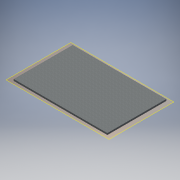
# Autodesk Inventor part: Zwischendecke
Saved by Autodesk Inventor 2017 (Build 210142000, 142)
## iProperties
Created: 2017-06-01
Part Number: Zwischendecke
Material: Beton
Document SubType Name: Modeling
Designer: Fake
Density: 2.40731 g/cm^3
Appearance: Waschbeton - warm-grau
Author: Fake
Autodesk Inventor part; units mm, degrees
ref_plane "YZ Plane" through (0, 0, 0) normal (1, 0, 0) x (0, 1, 0)
ref_plane "XZ Plane" through (0, 0, 0) normal (0, 1, 0) x (-1, 0, 0)
ref_plane "XY Plane" through (0, 0, 0) normal (0, 0, 1) x (1, 0, 0)
ref_plane "Arbeitsebene1" through (-317.6174, -149.9495, 3700) normal (0, 0, 1) x (1, 0, 0)
sketch "Skizze1" plane through (-317.6174, -149.9495, 3700) normal (0, 0, 1) x (1, 0, 0)
  line L0 (5797.6174, 3524.9495) -> (5797.6174, -3225.0505) projected
  line L1 (5797.6174, -3225.0505) -> (-3682.3826, -3225.0505) projected
  line L2 (-3682.3826, -3225.0505) -> (-3682.3826, -1925.0505) projected
  line L3 (-3682.3826, -1925.0505) -> (-5162.3826, -1925.0505) projected
  line L4 (-5162.3826, -1925.0505) -> (-5162.3826, 3524.9495) projected
  line L5 (-5162.3826, 3524.9495) -> (5797.6174, 3524.9495) projected
  line L6 (-5162.3826, -3425.0505) -> (-5162.3826, -2125.0505) projected
  line L7 (-5162.3826, -2125.0505) -> (-3882.3826, -2125.0505) projected
  line L8 (-3882.3826, -2125.0505) -> (-3882.3826, -3425.0505) projected
  line L9 (-3882.3826, -3425.0505) -> (5997.6174, -3425.0505) projected
  line L10 (5997.6174, -3425.0505) -> (5997.6174, 3724.9495) projected
  line L11 (5997.6174, 3724.9495) -> (-5362.3826, 3724.9495) projected
  line L12 (-5362.3826, 3724.9495) -> (-5362.3826, -3425.0505) projected
  line L13 (-5362.3826, -3425.0505) -> (-5162.3826, -3425.0505) projected
  line L14 (-5362.3826, 3724.9495) -> (5997.6174, 3724.9495)
  line L15 (5997.6174, 3724.9495) -> (5997.6174, -3425.0505)
  line L16 (5997.6174, -3425.0505) -> (-5362.3826, -3425.0505)
  line L17 (-5362.3826, -3425.0505) -> (-5362.3826, 3724.9495)
  constraints: 8 end point, 2 parallel, 1 horizontal, 1 perpendicular
extrude "Extrusion1" add sketch "Skizze1" along normal blind 200 contours L0 L1 L2 L3 L4 L5 | L13 L12 L11 L10 L9 L8 L7 L6 | L6 L7 L8 L16
